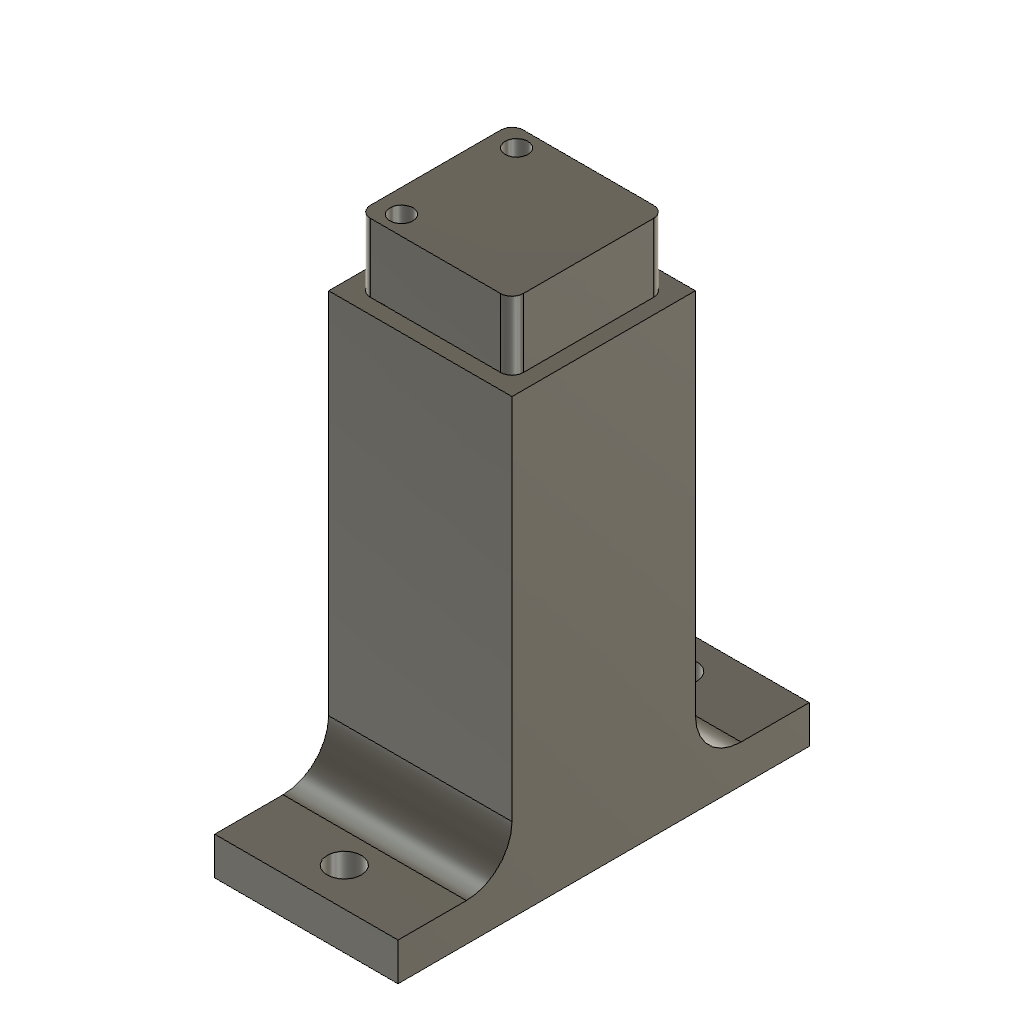
switch (Autodesk Fusion 360 design; units mm, degrees)
part number: 2026-09-25-20-23-26-193
Autodesk Fusion 360 part; units mm, degrees
sketch "Sketch1" plane through (0, 0, 0) normal (0, 0, 1) x (1, 0, 0)
  line L0 (8.575, -10.075) -> (-8.575, -10.075)
  line L1 (-10.075, -8.575) -> (-10.075, 8.575)
  line L2 (-8.575, 10.075) -> (8.575, 10.075)
  line L3 (10.075, 8.575) -> (10.075, -8.575)
  line L4 (10.075, -10.075) -> (-10.075, 10.075) construction
  line L5 (-10.075, -10.075) -> (10.075, 10.075) construction
  circle A0 centre (-6.975, 7.575) radius 1.5
  circle A1 centre (-6.975, -7.575) radius 1.5
  arc A2 (-8.575, 10.075) -> (-10.075, 8.575) centre (-8.575, 8.575) ccw
  arc A3 (-10.075, -8.575) -> (-8.575, -10.075) centre (-8.575, -8.575) ccw
  arc A4 (10.075, 8.575) -> (8.575, 10.075) centre (8.575, 8.575) ccw
  arc A5 (8.575, -10.075) -> (10.075, -8.575) centre (8.575, -8.575) ccw
  dimension "d1" = 20.15
  dimension "d2" = 20.15
  dimension "d3" = 3
  dimension "d4" = 3
  dimension "d5" = 2.5
  dimension "d6" = 3.1
  dimension "d7" = 2.5
  dimension "d8" = 3.1
  dimension "d9" = 1.5
  dimension "d10" = 1.5
  dimension "d11" = 1.5
  constraint horizontal L0
  constraint perpendicular L0 L1
  constraint parallel L0 L2
  constraint parallel L1 L3
  constraint coincident L4 origin
  constraint coincident L5 origin
  constraint coincident L4.end L1
  constraint coincident L4.end L2
  constraint tangent L1 A2
  constraint tangent L2 A2
  constraint coincident L5.start L0
  constraint coincident L5.start L1
  constraint tangent L0 A3
  constraint tangent L1 A3
  constraint coincident L5.end L2
  constraint coincident L5.end L3
  constraint tangent L2 A4
  constraint tangent L3 A4
  constraint coincident L4.start L0
  constraint coincident L4.start L3
  constraint tangent L0 A5
  constraint tangent L3 A5
  constraint equal A4 A5
  measures "d1" distance of L5.start L4.end
  measures "d2" distance of L4.end L5.end
  measures "d3" diameter of A0
  measures "d4" diameter of A1
  measures "d5" distance of L2 A0.centre
  measures "d6" distance of L1 A0.centre
  measures "d7" distance of L0 A1.centre
  measures "d8" distance of L1 A1.centre
  measures "d9" radius of A2
  measures "d10" radius of A3
  measures "d11" radius of A4
extrude "Extrude1" add sketch "Sketch1" along normal blind 9 makes body 1
extrude "Extrude2" add 1 faces at (4.8048, -2.2433, 0) along direction (0, 0, -1) blind 59.45 separate body on bodies 1 makes body 2
move_face "OffsetFaces1" offset 2 8 faces at (-10.075, -2.8583, -19.8167) (2.8583, -10.075, -19.8167) (-9.9676, -9.1325, -39.6333) (9.6606, -9.6101, -39.6333) (10.075, 2.8583, -19.8167) (9.7541, 9.5022, -39.6333) (-2.8583, 10.075, -19.8167) (-9.325, 9.874, -39.6333) on bodies 2
sketch "Sketch2" plane through (0, 0, 0) normal (0, 0, 1) x (-1, 0, 0)
  circle A0 centre (6.975, -7.575) radius 1.5
  circle A1 centre (6.975, 7.575) radius 1.5
  arc A2 (12.075, 8.575) -> (8.575, 12.075) centre (8.575, 8.575) ccw
  line L0 (8.575, 12.075) -> (-8.575, 12.075)
  arc A3 (-8.575, 12.075) -> (-12.075, 8.575) centre (-8.575, 8.575) ccw
  line L1 (-12.075, 8.575) -> (-12.075, -8.575)
  arc A4 (-12.075, -8.575) -> (-8.575, -12.075) centre (-8.575, -8.575) ccw
  line L2 (-8.575, -12.075) -> (8.575, -12.075)
  arc A5 (8.575, -12.075) -> (12.075, -8.575) centre (8.575, -8.575) ccw
  line L3 (12.075, -8.575) -> (12.075, 8.575)
  circle A6 centre (6.975, -7.575) radius 2.5
  circle A7 centre (6.975, 7.575) radius 2.5
  dimension "d17" = 5
  dimension "d18" = 5
  constraint concentric A0 A6
  constraint concentric A1 A7
  measures "d17" diameter of A6
  measures "d18" diameter of A7
delete_face "DeleteFace1" 2 faces at (-5.4825, -7.7244, -19.8167) (-5.4825, 7.4256, -19.8167) on bodies 2
extrude "Extrude3" cut sketch "Sketch2" against normal blind 5 contours A0 | A1 | A6 | A7 bodies 2
delete_face "DeleteFace2" 4 faces at (-12.071, 8.7415, -39.6333) (-8.7415, -12.071, -19.8167) (10.325, -11.6061, -39.6333) (8.7415, 12.071, -39.6333) on bodies 2
sketch "Sketch3" plane through (0, 0, -59.45) normal (0, 0, -1) x (1, 0, 0)
  line L0 (12.075, -12.075) -> (12.075, 12.075)
  line L1 (12.075, 12.075) -> (-12.075, 12.075)
  line L2 (-12.075, 12.075) -> (-12.075, -12.075)
  line L3 (-12.075, -12.075) -> (12.075, -12.075)
  line L4 (-12.075, 12.075) -> (12.075, 12.075)
  line L5 (12.075, 12.075) -> (12.075, 27.075)
  line L6 (12.075, 27.075) -> (-12.075, 27.075)
  line L7 (-12.075, 27.075) -> (-12.075, 12.075)
  line L8 (-12.075, -12.075) -> (12.075, -12.075)
  line L9 (12.075, -12.075) -> (12.075, -27.075)
  line L10 (12.075, -27.075) -> (-12.075, -27.075)
  line L11 (-12.075, -27.075) -> (-12.075, -12.075)
  dimension "d21" = 15
  dimension "d22" = 15
  constraint horizontal L4
  constraint vertical L5
  constraint horizontal L6
  constraint vertical L7
  constraint coincident L1.end L2.start
  constraint horizontal L8
  constraint vertical L9
  constraint horizontal L10
  constraint vertical L11
  constraint coincident L2.end L3.start
  measures "d21" distance of L1.end L6.end
  measures "d22" distance of L2.end L10.end
extrude "Extrude4" add sketch "Sketch3" against normal blind 5 contours L3 L8 L9 L10 L11 | L1 L4 L5 L6 L7 bodies 2
fillet "Fillet1" radius 6 2 edges at (0, -12.075, -54.45) (0, 12.075, -54.45) on bodies 2
sketch "Sketch4" plane through (0, 0, -54.45) normal (0, 0, 1) x (-1, 0, 0)
  line L0 (12.075, -18.075) -> (-12.075, -18.075)
  line L1 (-12.075, -18.075) -> (-12.075, -27.075)
  line L2 (-12.075, -27.075) -> (12.075, -27.075)
  line L3 (12.075, -27.075) -> (12.075, -18.075)
  circle A0 centre (0, -22.075) radius 2.25
  dimension "d27" = 4.5
  dimension "d28" = 5
  measures "d27" diameter of A0
  measures "d28" distance of L2 A0.centre
extrude "Extrude5" cut sketch "Sketch4" against normal blind 13 contours A0 bodies 2
ref_plane "WorkPlane1" through (0, 0, -24.225) normal (0, -1, 0) x (-1, 0, 0)
mirror "Mirror1" about plane through (0, 0, -24.225) normal (0, -1, 0) of "Extrude5"
